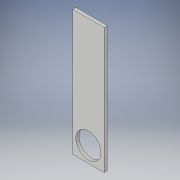
# Autodesk Inventor part: Verbindungsstück_Rolle
Saved by Autodesk Inventor 2018 (Build 220112000, 112)
## iProperties
Created: 2018-01-12
Part Number: Verbindungsstück_Rolle
Material: Generisch
Document SubType Name: Modeling
Designer: Julian
Density: 1 g/cm^3
Appearance: Vorgabe
Author: Julian
Autodesk Inventor part; units mm, degrees
ref_plane "YZ Plane" through (0, 0, 0) normal (1, 0, 0) x (0, 1, 0)
ref_plane "XZ Plane" through (0, 0, 0) normal (0, 1, 0) x (-1, 0, 0)
ref_plane "XY Plane" through (0, 0, 0) normal (0, 0, 1) x (1, 0, 0)
sketch "Skizze1" plane through (0, 0, 0) normal (0, 1, 0) x (-1, 0, 0)
  line L0 (0, 0) -> (-10, 0)
  line L1 (-10, 0) -> (-10, 40)
  line L2 (-10, 40) -> (0, 40)
  line L3 (0, 40) -> (0, 0)
  dimension "d0" = 10
  dimension "d1" = 40
  constraints: 8 end point, 2 parallel, 1 horizontal, 1 perpendicular
  measures "d0" distance of L1.end L2.end
  measures "d1" distance of L0.end L1.end
extrude "Extrusion1" add sketch "Skizze1" along normal blind 1
sketch "Skizze2" plane through (0, 0, 0) normal (0, -1, 0) x (1, 0, 0)
  line L0 (10, 0) -> (0, 0) projected
  line L1 (0, 0) -> (5, 0)
  line L2 (5, 0) -> (5, 5)
  dimension "d4" = 5
  constraints: 4 end point, 1 midpoint, 1 perpendicular
  measures "d4" distance of L1.end L2.end
hole "Bohrung1" at (5, 0, 5) direction (0, 1, 0) diameter 8 depth 8 tip angle 118
